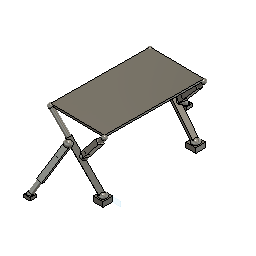
TT-1 (Autodesk Fusion 360 design; units mm, degrees)
Autodesk Fusion 360 part; units mm, degrees
note: some values were not read from the file. Chosen so that the rebuilt part matches the saved one: which bodies a step acts on.
sketch "Sketch1" plane through (0, 0, 0) normal (0, 1, 0) x (1, 0, 0)
  line L0 (5, -50) -> (-5, -50)
  line L1 (-5, -50) -> (-5, -40)
  line L2 (-5, -40) -> (5, -40)
  line L3 (5, -40) -> (5, -50)
  constraint horizontal L0
  constraint vertical L1
  constraint horizontal L2
  constraint vertical L3
extrude "Extrude1" add sketch "Sketch1" along normal blind 5 makes body 1
sketch "Sketch2" plane through (0, 0, 40) normal (0, 0, -1) x (-1, 0, 0)
  line L0 (-5, 0) -> (5, 0)
  line L1 (5, 0) -> (5, 5)
  line L2 (5, 5) -> (-5, 5)
  line L3 (-5, 5) -> (-5, 0)
sphere "SpherePrimitive1" cut diameter 8 placed x (-1, 0, 0) y (0, 0, 1) z (0, 1, 0) at (0, 5, 45) bodies 1
sketch "Sketch4" plane through (0, 0, 0) normal (0, 0, 1) x (1, 0, 0)
  line L0 (-10, 5) -> (-15, 5)
  line L1 (-15, 5) -> (-15, 50)
  line L2 (-15, 50) -> (-10, 50)
  line L3 (-10, 50) -> (-10, 5)
  constraint horizontal L0
  constraint vertical L1
  constraint horizontal L2
  constraint vertical L3
extrude "Extrude2" add sketch "Sketch4" against normal blind 5 separate body makes body 2
sphere "SpherePrimitive2" add diameter 8 placed x (1, 0, 0) y (0, 0, 1) z (0, -1, 0) at (-12.5, 5, -2.5) bodies 2
sketch "Sketch6" plane through (0, 50, 0) normal (0, 1, 0) x (-1, 0, 0)
  line L0 (15, 0) -> (10, 0)
  line L1 (10, 0) -> (10, -5)
  line L2 (10, -5) -> (15, -5)
  line L3 (15, -5) -> (15, 0)
  circle A0 centre (12.5, -2.5) radius 2.25
  dimension "d7" = 4.5
  measures "d7" diameter of A0
extrude "Extrude3" add sketch "Sketch6" along normal blind 45 separate body contours A0 makes body 3
sphere "SpherePrimitive3" add diameter 5 placed x (-1, 0, 0) y (0, 0, 1) z (0, 1, 0) at (-12.5, 95, -2.5) bodies 3
copy_body "CopyPasteBodies1" bodies 2 3 makes body 4 makes body 5
move_body "Move1" bodies 4 5 to x (1, 0, 0) y (0, 1, 0) z (0, 0, 1) at (2.5, 32.3956, 0)
move_body "Move2" bodies 5 4 to x (0.824267, -0.566201, 0) y (0.566201, 0.824267, 0) z (0, 0, 1) at (-22.9308, 0.9096, 0)
copy_body "CopyPasteBodies2" bodies 4 makes body 6
move_body "Move3" bodies 6 to x (1, 0, 0) y (0, 1, 0) z (0, 0, 1) at (0, 0, 0)
combine "Combine1" operation cut target body 2 tool bodies 6
extrude "Extrude4" cut 1 faces at (14.7922, 74.9595, -3.3333) along direction (-0.566201, -0.824267, 0) blind 10 on bodies 4 bodies 4
extrude "Extrude5" cut 1 faces at (14.2431, 75.3367, -3.0134) along direction (0.566201, 0.824267, 0) blind 10 on bodies 5 bodies 5
move_body "Move4" bodies 5 to x (1, 0, 0) y (0, 1, 0) z (0, 0, 1) at (-12.4628, -18.1432, 0)
extrude "Extrude6" add 1 faces at (-13.3333, 50, -1.6667) along direction (0, 1, 0) blind 5 on bodies 2 bodies 2
extrude "Extrude7" add 1 faces at (-13.0979, 50, -3.5089) along direction (0, -1, 0) blind 5 on bodies 3 bodies 3
move_body "Move5" bodies 3 to x (1, 0, 0) y (0, 1, 0) z (0, 0, 1) at (0, 8.1325, 0)
copy_body "CopyPasteBodies3" bodies 5 4 makes body 7 makes body 8
move_body "Move6" bodies 7 8 to x (-1, 0, 0) y (0, -1, 0) z (0, 0, 1) at (-25, 88.5686, 0)
move_body "Move7" bodies 7 8 to x (0.97619, -0.216915, 0) y (0.216915, 0.97619, 0) z (0, 0, 1) at (-11.4573, -2.5051, 0)
copy_body "CopyPasteBodies4" bodies 8 makes body 9
combine "Combine2" operation cut target body 2 tool bodies 9
copy_body "CopyPasteBodies5" bodies 1 makes body 10
move_body "Move8" bodies 10 to x (1, 0, 0) y (0, 1, 0) z (0, 0, 1) at (0, 0, -15.2448)
scale "Scale1" factor 0.625 about (5, 5, 24.7552) bodies 10
move_body "Move9" bodies 10 to x (1, 0, 0) y (0, 1, 0) z (0, 0, 1) at (0, 4.3642, 5.1625)
move_body "Move10" bodies 10 to x (1, 0, 0) y (0, 1, 0) z (0, 0, 1) at (1.25, -6.2392, 10.0823)
move_body "Move11" bodies 10 to x (1, 0, 0) y (0, 1, 0) z (0, 0, 1) at (0, 0, -13.3948)
move_body "Move12" bodies 7 8 to x (0.965133, 0.040512, 0.258607) y (-0.039132, 0.999179, -0.010485) z (-0.258819, 0, 0.965926) at (0.8141, 0.6493, 4.3256)
move_body "Move13" bodies 5 4 to x (0.913545, 0, -0.406737) y (0, 1, 0) z (0.406737, 0, 0.913545) at (0.1523, 0, -4.2835)
move_body "Move14" bodies 7 3 2 5 4 8 to x (0.906308, 0, 0.422618) y (0, 1, 0) z (-0.422618, 0, 0.906308) at (-3.2842, 0, 4.8143)
move_body "Move15" bodies 4 8 2 3 7 5 to x (1, 0, 0) y (0, 1, 0) z (0, 0, 1) at (4.6922, 0, -41.6046)
move_body "Move16" bodies 1 to x (1, 0, 0) y (0, 1, 0) z (0, 0, 1) at (-8.8643, 0, -89.3388)
move_body "Move17" bodies 10 to x (1, 0, 0) y (0, 1, 0) z (0, 0, 1) at (-50.2972, 0.0198, -105.3684)
mirror "Mirror1" about plane through (0, 0, 0) normal (0, 0, 1) of bodies 10 1 3 2 4 8 5 7 makes body 11 at (-7.1976, 0, 42.6721) makes body 12 at (-11.6157, 30.4247, 42.8633) makes body 13 at (-10.9266, 72.7692, 43.439) makes body 14 at (-3.0205, 35.7707, 42.5356) makes body 15 at (25.1583, 83, 40.5118) makes body 16 at (-39.1915, 10.0755, 71.0443) makes body 17 at (-14.0562, 52.9386, 46.9576) makes body 18 at (-44.6936, 2.8185, 75.6383)
move_body "Move18" bodies 3 13 to x (1, 0, 0) y (0, 1, 0) z (0, 0, 1) at (0, -9.1842, 0)
sketch "Sketch8" plane through (0, 0, 0) normal (0, 1, 0) x (1, 0, 0)
  line L0 (40, 50) -> (-15, 50)
  line L1 (-15, 50) -> (-15, -50)
  line L2 (-15, -50) -> (40, -50)
  line L3 (40, -50) -> (40, 50)
  constraint horizontal L0
  constraint vertical L1
  constraint horizontal L2
  constraint vertical L3
extrude "Extrude8" add sketch "Sketch8" along normal blind 2 separate body makes body 19
move_body "Move19" bodies 19 to x (1, 0, 0) y (0, 1, 0) z (0, 0, 1) at (0, 95.9987, 0)
copy_body "Body->Comp1" bodies 19 removing the originals makes body 20 in component "FLAT"
copy_body "Body->Comp2" bodies 1 removing the originals makes body 21 in component "L-main-fix"
copy_body "Body->Comp3" bodies 3 removing the originals makes body 22 in component "L-main-act"
copy_body "Body->Comp4" bodies 11 removing the originals makes body 23 in component "R-main-fix"
copy_body "Body->Comp5" bodies 13 removing the originals makes body 24 in component "R-main-act"
copy_body "Body->Comp6" bodies 14 removing the originals makes body 25 in component "R-high-base"
copy_body "Body->Comp7" bodies 15 removing the originals makes body 26 in component "R-high-act"
copy_body "Body->Comp8" bodies 10 removing the originals makes body 27 in component "L-low-fix"
copy_body "Body->Comp9" bodies 12 removing the originals makes body 28 in component "R-main-base"
copy_body "Body->Comp10" bodies 18 removing the originals makes body 29 in component "R-low-fix"
copy_body "Body->Comp11" bodies 2 removing the originals makes body 30 in component "L-main-base"
copy_body "Body->Comp12" bodies 4 removing the originals makes body 31 in component "L-high-base"
copy_body "Body->Comp13" bodies 8 removing the originals makes body 32 in component "L-low-base"
copy_body "Body->Comp14" bodies 5 removing the originals makes body 33 in component "L-high-act"
copy_body "Body->Comp15" bodies 16 removing the originals makes body 34 in component "R-low-act"
copy_body "Body->Comp16" bodies 7 removing the originals makes body 35 in component "L-low-act"
copy_body "Body->Comp17" bodies 17 removing the originals makes body 36 in component "R-low-base"
sketch "Sketch9" plane through (0, 0, 0) normal (0, 1, 0) x (1, 0, 0)
  line L0 (10, -60) -> (-60, -60)
  line L1 (-60, -60) -> (-60, 60)
  line L2 (-60, 60) -> (10, 60)
  line L3 (10, 60) -> (10, -60)
  constraint horizontal L0
  constraint vertical L1
  constraint horizontal L2
  constraint vertical L3
extrude "Extrude9" add sketch "Sketch9" along normal blind 81.626 separate body makes body 37
component "FLAT" placed x (0.999649, -0.004123, 0.026181) y (0.004117, 0.999991, 0.000289) z (-0.026182, -0.000181, 0.999657) at (-40.2712, -12.5801, -1.1343)
component "L-main-fix" placed x (0.999942, -0.000776, -0.010731) y (0.000951, 0.999866, 0.016351) z (0.010717, -0.01636, 0.999809) at (0.2833, -0.6092, -5.7937)
component "L-main-act" placed x (0.030348, -0.002341, -0.999537) y (-0.493807, 0.869405, -0.01703) z (0.869042, 0.494095, 0.025229) at (31.632, 23.6964, -57.6238)
component "R-main-fix" placed x (1, 0, 0) y (0, 1, 0) z (0, 0, 1) at (0, 0, 0)
component "R-main-act" placed x (0.68791, 0.445072, -0.573316) y (-0.515838, 0.855493, 0.045187) z (0.510579, 0.264654, 0.818087) at (-24.2583, -4.6908, 2.8833)
component "R-high-base" placed x (-0.458194, 0.868256, -0.190238) y (0.83032, 0.494486, 0.257006) z (0.317217, -0.040199, -0.947501) at (-72.3596, 22.4206, 73.7831)
component "R-high-act" placed x (-0.458194, 0.868256, -0.190238) y (0.83032, 0.494486, 0.257006) z (0.317217, -0.040199, -0.947501) at (-77.6858, 11.0642, 72.35)
component "L-low-fix" placed x (0.999934, 0.011499, 0.000859) y (-0.011517, 0.999611, 0.025411) z (-0.000567, -0.025419, 0.999677) at (-2.429, -1.1396, -5.1245)
component "R-main-base" placed x (0.68791, 0.445072, -0.573316) y (-0.515838, 0.855493, 0.045187) z (0.510579, 0.264654, 0.818087) at (-22.8257, -7.0667, 2.7578)
component "R-low-fix" placed x (1, 0.000458, -0.000579) y (-0.000457, 0.999999, 0.001328) z (0.00058, -0.001328, 0.999999) at (-2.3567, 0.0538, 1.9822)
component "L-main-base" placed x (0.030348, -0.002341, -0.999537) y (-0.493807, 0.869405, -0.01703) z (0.869042, 0.494095, 0.025229) at (32.2194, 22.6622, -57.6036)
component "L-high-base" placed x (-0.461682, 0.864633, 0.198139) y (0.873888, 0.481672, -0.065667) z (-0.152216, 0.142834, -0.977972) at (-66.3754, 27.6791, -91.3026)
component "L-low-base" placed x (0.964316, 0.2479, 0.092947) y (-0.258513, 0.957426, 0.128479) z (-0.05714, -0.147922, 0.987347) at (-11.3599, -8.1601, -9.1462)
component "L-high-act" placed x (-0.461682, 0.864633, 0.198139) y (0.873888, 0.481672, -0.065667) z (-0.152216, 0.142834, -0.977972) at (-71.9964, 16.7685, -91.8971)
component "R-low-act" placed x (0.836158, 0.510439, 0.200728) y (-0.423525, 0.833406, -0.355052) z (-0.34852, 0.211866, 0.913043) at (17.9848, 9.3499, 18.5693)
component "L-low-act" placed x (0.964316, 0.2479, 0.092947) y (-0.258513, 0.957426, 0.128479) z (-0.05714, -0.147922, 0.987347) at (-7.2737, 1.693, -1.3968)
component "R-low-base" placed x (0.836158, 0.510439, 0.200728) y (-0.423525, 0.833406, -0.355052) z (-0.34852, 0.211866, 0.913043) at (13.1428, -2.8229, 27.3558)
hidden bodies 37
equation "d19 = 5 / 8"
named bodies: "L-main-fix", "L-main-base", "L-main-act", "L-high-base", "L-high-act", "L-main-base (1)", "L-main-base (1) (1)", "L-main-act (1)", "L-low-act", "L-low-base", "L-main-base (1) (1) (1)", "L-fix", "L-low-fix", "R-main-fix", "R-main-base", "R-main-act", "R-high-base", "R-high-act", "R-low-act", "R-low-base", "R-low-fix", "FLAT"
